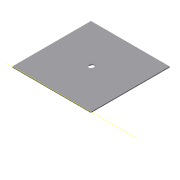
# Autodesk Inventor part: 00_coverslip
Saved by Autodesk Inventor 2019.4 (Build 234330000, 330)
## iProperties
Created: 2021-01-25
Part Number: 00_coverslip
Material: Generic
Document SubType Name: Modeling
Designer: diederichbenedict
Density: 1 g/cm^3
Appearance: Default
Author: diederichbenedict
Autodesk Inventor part; units mm, degrees
ref_plane "YZ Plane" through (0, 0, 0) normal (1, 0, 0) x (0, 1, 0)
ref_plane "XZ Plane" through (0, 0, 0) normal (0, 1, 0) x (-1, 0, 0)
ref_plane "XY Plane" through (0, 0, 0) normal (0, 0, 1) x (1, 0, 0)
sketch "Sketch1" plane through (0, 0, 0) normal (0, 1, 0) x (-1, 0, 0)
  line L0 (-9, -9) -> (9, -9)
  line L1 (9, -9) -> (9, 9)
  line L2 (9, 9) -> (-9, 9)
  line L3 (-9, 9) -> (-9, -9)
  line L4 (-9, -9) -> (9, 9) construction
  line L5 (9, -9) -> (-9, 9) construction
  point P0 (0, 0)
  dimension "d0" = 18
  dimension "d1" = 18
  constraints: 12 end point, 2 midpoint, 2 parallel, 1 horizontal, 1 perpendicular
  measures "d0" distance of L2.end L1.end
  measures "d1" distance of L1.end L0.end
extrude "Extrusion1" add sketch "Sketch1" along normal blind 0.2
ref_plane "Work Plane1" through (-9, 0.2, 9) normal (0, -0.7071, 0.7071) x (1, 0, 0)
sketch "Sketch2" plane through (-9, 0.2, 9) normal (0, -0.7071, 0.7071) x (1, 0, 0)
  line L0 (18, -12.8693) -> (0, -12.8693) projected
  line L1 (18, -0.1414) -> (18, -12.8693) projected
  line L2 (0, -0.1414) -> (18, -0.1414) projected
  line L3 (0, -12.8693) -> (0, -0.1414) projected
  circle A0 centre (9, -6.5054) radius 0.5
  dimension "d4" = 1
  constraints: 1 centre point, 1 coincident
  measures "d4" diameter of A0
extrude "Extrusion2" cut sketch "Sketch2" against normal through all contours A0
ref_plane "Work Plane2" through (-9, 0.2, 9) normal (0, 0.7071, 0.7071) x (-1, 0, 0)
sketch "Sketch3" plane through (-9, 0.2, 9) normal (0, 0.7071, 0.7071) x (-1, 0, 0)
  circle A0 centre (-9, -6.5054) radius 0.5 projected
  line L0 (-18, -12.7279) -> (0, -12.7279) projected
  line L1 (0, -12.7279) -> (0, 0) projected
  line L2 (0, 0) -> (-18, 0) projected
  line L3 (-18, 0) -> (-18, -12.7279) projected
  circle A1 centre (-9, -6.2225) radius 0.5
  dimension "d7" = 1
  constraints: 1 centre point, 1 coincident
  measures "d7" diameter of A1
extrude "Extrusion3" cut sketch "Sketch3" against normal through all contours A1 A0 | A0 A1 picked at (-9.0194, -6.2456) picked at (-9.0263, -5.8205)
body "Solid1"
